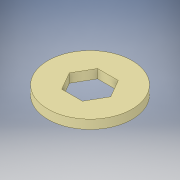
# Autodesk Inventor part: BASE_SOST.PERNO
Saved by Autodesk Inventor 2019 (Build 230136000, 136)
## iProperties
Created: 2020-02-12
Part Number: BASE_SOST.PERNO
Material: Genérico
Document SubType Name: Modeling
Designer: omar-
Density: 1 g/cm^3
Appearance: Valor por defecto
Author: omar-
Autodesk Inventor part; units mm, degrees
ref_plane "YZ Plane" through (0, 0, 0) normal (1, 0, 0) x (0, 1, 0)
ref_plane "XZ Plane" through (0, 0, 0) normal (0, 1, 0) x (-1, 0, 0)
ref_plane "XY Plane" through (0, 0, 0) normal (0, 0, 1) x (1, 0, 0)
sketch "Boceto1" plane through (0, 0, 0) normal (0, 1, 0) x (-1, 0, 0)
  line L0 (7.3901, 0) -> (3.695, -6.4)
  line L1 (3.695, -6.4) -> (-3.695, -6.4)
  line L2 (-3.695, -6.4) -> (-7.3901, 0)
  line L3 (-7.3901, 0) -> (-3.695, 6.4)
  line L4 (-3.695, 6.4) -> (3.695, 6.4)
  line L5 (3.695, 6.4) -> (7.3901, 0)
  circle A0 centre (0, 0) radius 15
  dimension "d0" = 12.8
  dimension "d1" = 0
  dimension "d2" = 30
  constraints: 12 end point, 2 coincident, 1 centre point, 13 other
  measures "d0" distance between parallel lines of L3 L0
  measures "d1" vertical distance of L0.start point (0, 0)
  measures "d2" diameter of A0
extrude "Extrusión1" add sketch "Boceto1" along normal blind 3.18
